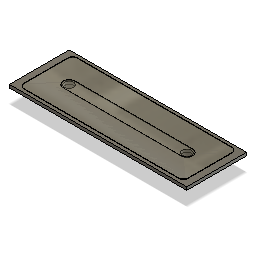
be1215d4-c3ec-41a3-ab22-ad0e6fc781e9 (Autodesk Fusion 360 design; units mm, degrees)
Autodesk Fusion 360 part; units mm, degrees
note: some values were not read from the file. Chosen so that the rebuilt part matches the saved one: which face or edge a step refers to. Set by a fixed rule: which sketch regions a step uses.
sketch "Sketch1" plane through (0, 0, 0) normal (0, 1, 0) x (1, 0, 0)
  line L0 (-45.2824, 41.5395) -> (30.3676, 41.5395)
  line L1 (30.3676, 41.5395) -> (30.3676, 16.0395)
  line L2 (30.3676, 16.0395) -> (-45.2824, 16.0395)
  line L3 (-45.2824, 16.0395) -> (-45.2824, 41.5395)
  circle A0 centre (-32.5574, 28.7895) radius 1.92
  circle A1 centre (17.6426, 28.7895) radius 1.92
  circle A2 centre (-32.5574, 28.7895) radius 3.15
  circle A3 centre (17.6426, 28.7895) radius 3.15
  line L4 (-32.5574, 28.7895) -> (-31.8105, 30.5583)
  line L5 (-32.5574, 41.5395) -> (-32.5574, 28.7895)
  line L6 (-32.5574, 28.7895) -> (-32.5574, 16.0395)
  line L7 (17.6426, 28.7895) -> (17.6426, 41.5395)
  line L8 (17.6426, 28.7895) -> (17.6426, 16.0395)
  line L9 (-32.5574, 28.7895) -> (-45.2824, 28.7895)
  line L10 (17.6426, 28.7895) -> (30.3676, 28.7895)
  line L11 (20.7926, 28.7895) -> (-35.7074, 28.7895) construction
  dimension "d1" = 75.65
  dimension "d2" = 25.5
  dimension "d5" = 3.84
  dimension "d6" = 3.84
  dimension "d7" = 6.3
  dimension "d8" = 6.3
  dimension "d31" = 56.5
  dimension "d33" = 50.5
  constraint horizontal L0
  constraint vertical L1
  constraint horizontal L2
  constraint vertical L3
  constraint concentric A0 A2
  constraint concentric A1 A3
  constraint coincident A0.centre A2.centre
  constraint coincident A0 L4.end
  constraint coincident L0 L5.start
  constraint perpendicular L0 L5
  constraint coincident L2 L6.end
  constraint perpendicular L2 L6
  constraint coincident A1.centre A3.centre
  constraint coincident L0 L7.end
  constraint perpendicular L0 L7
  constraint coincident L2 L8.end
  constraint perpendicular L2 L8
  constraint equal L7 L8
  constraint equal L6 L8
  constraint midpoint L3 L9.end
  constraint midpoint L1 L10.end
  constraint equal L9 L10
  constraint coincident A3 L11.start
  constraint coincident L10 L11.start
  constraint coincident A2 L11.end
  constraint coincident L9 L11.end
  constraint parallel L9 L11
  measures "d1" distance of L0.start L0.end
  measures "d2" distance of L0.start L2.end
  measures "d5" diameter of A0
  measures "d6" diameter of A1
  measures "d7" diameter of A2
  measures "d8" diameter of A3
  measures "d31" distance of L11.start L11.end
extrude "Extrude1" add sketch "Sketch1" against normal blind 1.32 makes body 1
sketch "Sketch2" plane through (0, 0, 0) normal (0, 0, 1) x (1, 0, 0)
  line L0 (-13.3564, 21.7967) -> (-7.3564, 21.7967)
  line L1 (-13.1564, 27.7894) -> (-7.5565, 27.8041)
  line L2 (-13.1564, 27.7894) -> (-13.3564, 21.7967)
  line L3 (-7.5565, 27.8041) -> (-7.3564, 21.7967)
  line L4 (-12.4564, 27.7967) -> (-8.2564, 27.7967)
  line L5 (-12.2764, 21.7967) -> (-8.4364, 21.7967)
  line L6 (-12.4564, 27.7967) -> (-12.2764, 21.7967)
  line L7 (-8.2564, 27.7967) -> (-8.4364, 21.7967)
  line L8 (-10.3564, 21.7967) -> (-10.3564, 27.7967)
  dimension "d11" = 6
  dimension "d12" = 5.6
  dimension "d14" = 4.2
  dimension "d15" = 3.84
  constraint horizontal L0
  constraint horizontal L4
  constraint horizontal L5
  constraint midpoint L5 L8.start
  constraint midpoint L4 L8.end
  constraint perpendicular L4 L8
  measures "d11" distance of L0.start L0.end
  measures "d12" distance of L1.start L1.end
  measures "d14" distance of L4.start L4.end
  measures "d15" distance of L5.end L5.start
revolve "Revolve1" add sketch "Sketch2" angle 360 about axis through (-10.3564, 21.7967, 0) along (0, 1, 0) separate body contours L0 L1 L2 L6 makes body 2
move_body "Move1" bodies 2 to x (1, 0, 0) y (0, 1, 0) z (0, 0, 1) at (27.999, -21.7967, -28.7895)
copy_body "CopyPasteBodies1" bodies 2 makes body 3
move_body "Move2" bodies 3 to x (1, 0, 0) y (0, 1, 0) z (0, 0, 1) at (-50.2, 0, 0)
sketch "Sketch3" plane through (0, 0, 0) normal (0, 1, 0) x (1, 0, 0)
  line L0 (-32.5574, 31.2895) -> (17.6426, 31.2895)
  line L1 (17.6426, 31.2895) -> (17.6426, 26.2895)
  line L2 (17.6426, 26.2895) -> (-32.5574, 26.2895)
  line L3 (-32.5574, 26.2895) -> (-32.5574, 31.2895)
  circle A0 centre (17.6426, 28.7895) radius 2.5
  circle A1 centre (-32.5574, 28.7895) radius 2.5
  point P0 (-32.5574, 28.7895)
  point P1 (17.6426, 28.7895)
  dimension "d18" = 5
  dimension "d32" = 5
  constraint horizontal L0
  constraint vertical L1
  constraint horizontal L2
  constraint vertical L3
  constraint coincident L0.end A0
  constraint midpoint L3 P0
  constraint coincident L0.start A1
  constraint tangent L0 A1
  constraint coincident P0 A1.centre
  constraint coincident P1 A0.centre
  measures "d18" distance of L0.start L2.end
  measures "d32" diameter of A0
extrude "Extrude2" cut sketch "Sketch3" against normal blind 0.2 contours L0 L2 A0 A1 bodies 1
extrude "Extrude3" cut sketch "Sketch3" against normal blind 0.2 contours L3 A1 | L3 A1 | L1 A0 | L1 A0 bodies 1
mirror "Mirror1" about plane through (0, 0, 0) normal (0, 1, 0) of bodies 3 2 makes body 4 at (-33.2176, -0.9988, -25.8972) makes body 5 at (16.1592, -0.9988, -26.2203)
move_body "Move3" bodies 4 5 to x (1, 0, 0) y (0, 1, 0) z (0, 0, 1) at (0, -1.32, 0)
extrude "Extrude4" cut sketch "Sketch1" against normal blind 1.5 contours A0 L5 L9 | A0 L4 L5 | A0 L6 L9 | A1 L7 L8 | A1 L7 L10 | A0 L4 L6 | A1 L8 L10 bodies 1
sketch "Sketch4" plane through (0, 0, 0) normal (0, 1, 0) x (-1, 0, 0)
  line L0 (45.2824, -16.0395) -> (-30.3676, -16.0395)
  line L1 (-30.3676, -16.0395) -> (-30.3676, -41.5395)
  line L2 (-30.3676, -41.5395) -> (45.2824, -41.5395)
  line L3 (45.2824, -41.5395) -> (45.2824, -16.0395)
  arc A0 (-17.6426, -26.2895) -> (-17.6426, -31.2895) centre (-17.6426, -28.7895) ccw
  line L4 (-17.6426, -26.2895) -> (32.5574, -26.2895)
  arc A1 (32.5574, -31.2895) -> (32.5574, -26.2895) centre (32.5574, -28.7895) ccw
  line L5 (32.5574, -31.2895) -> (-17.6426, -31.2895)
  line L6 (40.4574, -40.1645) -> (-25.5426, -40.1645)
  line L7 (-27.5426, -38.1645) -> (-27.5426, -19.4145)
  line L8 (-25.5426, -17.4145) -> (40.4574, -17.4145)
  line L9 (42.4574, -19.4145) -> (42.4574, -38.1645)
  line L10 (7.4574, -40.1645) -> (7.4574, -41.5395)
  line L11 (42.4574, -28.7895) -> (45.2824, -28.7895)
  arc A2 (-27.5426, -38.1645) -> (-25.5426, -40.1645) centre (-25.5426, -38.1645) ccw
  arc A3 (-25.5426, -17.4145) -> (-27.5426, -19.4145) centre (-25.5426, -19.4145) ccw
  arc A4 (42.4574, -19.4145) -> (40.4574, -17.4145) centre (40.4574, -19.4145) ccw
  arc A5 (40.4574, -40.1645) -> (42.4574, -38.1645) centre (40.4574, -38.1645) ccw
  point P0 (42.4574, -40.1645)
  point P1 (-27.5426, -40.1645)
  point P2 (42.4574, -17.4145)
  dimension "d26" = 70
  dimension "d27" = 22.75
  dimension "d28" = 2
  constraint horizontal L6
  constraint vertical L7
  constraint horizontal L8
  constraint vertical L9
  constraint midpoint L2 L10.end
  constraint midpoint L3 L11.end
  constraint perpendicular L6 L10
  constraint perpendicular L9 L11
  constraint coincident L6 L10.start
  constraint coincident P1 L6
  constraint coincident P1 L7
  constraint tangent L6 A2
  constraint tangent L7 A2
  constraint tangent L7 A3
  constraint tangent L8 A3
  constraint equal A2 A3
  constraint coincident P2 L8
  constraint coincident L9 L11.start
  constraint coincident P2 L9
  constraint tangent L8 A4
  constraint tangent L9 A4
  constraint equal A2 A4
  constraint coincident P0 L9
  constraint coincident P0 L6
  constraint tangent L9 A5
  constraint tangent L6 A5
  constraint equal A2 A5
  measures "d26" distance of P0 P1
  measures "d27" distance of P0 P2
  measures "d28" radius of A2
extrude "Extrude5" add sketch "Sketch4" along normal blind 0.18 separate body contours L6 L7 L8 L9 A2 A3 A4 A5 | A0 L4 A1 L5 makes body 6
delete_body "RemoveBody1" bodies 2
delete_body "RemoveBody2" bodies 3
